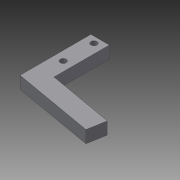
# Autodesk Inventor part: Swinging2
Saved by Autodesk Inventor 2015 (Build 190159000, 159)
## iProperties
Created: 2017-03-28
Part Number: Swinging2
Material: Generic
Document SubType Name: Modeling
Designer: Guy
Density: 1 g/cm^3
Appearance: Default
Author: Guy
Autodesk Inventor part; units mm, degrees
ref_plane "YZ Plane" through (0, 0, 0) normal (1, 0, 0) x (0, 1, 0)
ref_plane "XZ Plane" through (0, 0, 0) normal (0, 1, 0) x (-1, 0, 0)
ref_plane "XY Plane" through (0, 0, 0) normal (0, 0, 1) x (1, 0, 0)
sketch "Sketch1" plane through (0, 0, 0) normal (0, 0, 1) x (1, 0, 0)
  line L0 (0, 0) -> (15, 0)
  line L1 (15, 0) -> (15, -45)
  line L2 (15, -45) -> (67.6047, -54.2756)
  line L3 (67.6047, -54.2756) -> (65, -69.0477)
  line L4 (65, -69.0477) -> (0, -57.5865)
  line L5 (0, -57.5865) -> (0, 0)
  dimension "d1" = 15
  dimension "d2" = 45
  dimension "d3" = 15
  dimension "d4" = 100
  dimension "d5" = 65
  constraints: 12 end point, 3 perpendicular, 1 horizontal, 1 parallel
  measures "d1" distance of L0.start L0.end
  measures "d2" distance of L0.end L1.end
  measures "d3" distance of L2.end L3.end
  measures "d4" angle of L2 L1
  measures "d5" distance from line of L5 L3.end
extrude "Extrusion1" add sketch "Sketch1" along normal blind 10
sketch "Sketch2" plane through (0, 0, 10) normal (0, 0, 1) x (1, 0, 0)
  circle A0 centre (7.5, -5) radius 2.5
  circle A1 centre (7.5, -30) radius 2.5
  line L0 (15, 0) -> (0, 0) projected
  line L1 (0, 0) -> (0, -57.5865) projected
  dimension "d8" = 5
  dimension "d9" = 5
  dimension "d10" = 5
  dimension "d11" = 7.5
  dimension "d12" = 7.5
  dimension "d13" = 30
  constraints: 2 centre point
  measures "d8" diameter of A0
  measures "d9" diameter of A1
  measures "d10" distance from line of A0.centre L0
  measures "d11" distance from line of A0.centre L1
  measures "d12" distance from line of L1 A1.centre
  measures "d13" distance from line of L0 A1.centre
extrude "Extrusion2" cut sketch "Sketch2" against normal up to next
equation "\"d12\" = d11"
body "Solid1"
